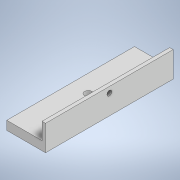
# Autodesk Inventor part: Угольник-10
Saved by Autodesk Inventor 2022 (Build 260153000, 153)
## iProperties
Created: 2021-12-03
Part Number: Угольник-10
Material: Типовые
Document SubType Name: Modeling
Designer: Украинцев
Density: 1 g/cm^3
Appearance: По умолчанию
Author: Украинцев
Autodesk Inventor part; units mm, degrees
ref_plane "YZ Plane" through (0, 0, 0) normal (1, 0, 0) x (0, 1, 0)
ref_plane "XZ Plane" through (0, 0, 0) normal (0, 1, 0) x (-1, 0, 0)
ref_plane "XY Plane" through (0, 0, 0) normal (0, 0, 1) x (1, 0, 0)
sketch "Эскиз1" plane through (0, 0, 0) normal (0, 1, 0) x (-1, 0, 0)
  line L0 (-44, 145) -> (44, 145)
  line L1 (44, 145) -> (44, -145)
  line L2 (44, -145) -> (-44, -145)
  line L3 (-44, -145) -> (-44, 145)
  line L4 (-44, 145) -> (44, -145) construction
  line L5 (44, 145) -> (-44, -145) construction
  line L6 (44, 0) -> (4, 0)
  circle A0 centre (4, 0) radius 8.5
  point P0 (0, 0)
  dimension "d0" = 88
  dimension "d1" = 290
  dimension "d2" = 40
  dimension "d3" = 17
  constraints: 14 end point, 3 midpoint, 2 horizontal, 2 parallel, 1 centre point, 1 coincident, 1 perpendicular
  measures "d0" distance of L1.end L2.end
  measures "d1" distance of L0.end L1.end
  measures "d2" distance of L6.start L6.end
  measures "d3" diameter of A0
extrude "Выдавливание1" add sketch "Эскиз1" along normal blind 20
sketch "Эскиз2" plane through (44, 0, 145) normal (1, 0, 0) x (0, 0, -1)
  line L0 (0, 0) -> (290, 0)
  line L1 (290, 0) -> (290, 58)
  line L2 (290, 58) -> (0, 58)
  line L3 (0, 58) -> (0, 0)
  line L4 (0, 58) -> (145, 58)
  line L5 (145, 58) -> (145, 45)
  circle A0 centre (145, 45) radius 5.5
  point P0 (145, 0)
  dimension "d6" = 58
  dimension "d7" = 145
  dimension "d8" = 13
  dimension "d9" = 11
  constraints: 12 end point, 2 parallel, 2 perpendicular, 1 centre point, 1 coincident, 1 horizontal, 1 midpoint
  measures "d6" distance of L1.end L0.end
  measures "d7" distance of L2.end L4.end
  measures "d8" distance of L4.end L5.end
  measures "d9" diameter of A0
extrude "Выдавливание2" add sketch "Эскиз2" against normal blind 8
